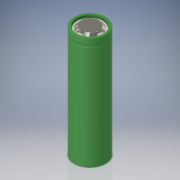
# Autodesk Inventor part: Battery18650
Saved by Autodesk Inventor 2017 (Build 210142000, 142)
## iProperties
Manager: Bradley
Company: Zetta & Zepto Technology
Created: 2016-08-15
Part Number: Battery18650
Material: Stainless Steel
Document SubType Name: Modeling
Designer: Bradley
Mass: 47 g
Surface Area: 43.2617 cm^2
Volume: 16.9329 cm^3
Density: 2.77566 g/cm^3
Appearance: Smooth - Dark Forest Green
Author: Bradley
Autodesk Inventor part; units mm, degrees
ref_plane "YZ Plane" through (0, 0, 0) normal (1, 0, 0) x (0, 1, 0)
ref_plane "XZ Plane" through (0, 0, 0) normal (0, 1, 0) x (-1, 0, 0)
ref_plane "XY Plane" through (0, 0, 0) normal (0, 0, 1) x (1, 0, 0)
sketch "Sketch1" plane through (0, 0, 0) normal (0, 0, 1) x (1, 0, 0)
  line L0 (0, 32.5) -> (0, -32.5)
  line L1 (9.15, -32.15) -> (9.15, 27.3)
  line L2 (9.15, 29.3) -> (9.15, 32)
  line L3 (8.85, 32.3) -> (7.95, 32.3)
  line L4 (7.65, 32) -> (7.65, 31.3)
  line L5 (7.35, 31) -> (6.65, 31)
  line L6 (6.65, 31) -> (5.2379, 32.4121)
  line L7 (5.0257, 32.5) -> (0, 32.5)
  arc A0 (8.85, -32.45) -> (9.15, -32.15) centre (8.85, -32.15) ccw
  arc A1 (9.15, 27.3) -> (9.0674, 27.5752) centre (8.65, 27.3) ccw
  arc A2 (9.0674, 29.0248) -> (9.15, 29.3) centre (8.65, 29.3) ccw
  arc A3 (9.15, 32) -> (8.85, 32.3) centre (8.85, 32) ccw
  arc A4 (5.2379, 32.4121) -> (5.0257, 32.5) centre (5.0257, 32.2) ccw
  arc A5 (7.95, 32.3) -> (7.65, 32) centre (7.95, 32) ccw
  arc A6 (7.35, 31) -> (7.65, 31.3) centre (7.35, 31.3) ccw
  arc A7 (9.0674, 29.0248) -> (9.0674, 27.5752) centre (10.1667, 28.3) ccw
  line L8 (8.85, -32.45) -> (8, -32.45)
  line L9 (0, -32.5) -> (8, -32.5)
  line L10 (8, -32.5) -> (8, -32.45)
  point P0 (0, 0)
  point P1 (9.15, 32.3)
  point P2 (7.65, 32.3)
  point P3 (7.65, 31)
  point P4 (0, 0)
  dimension "d0" = 65
  dimension "d1" = 18.3
  dimension "d2" = 0.2
  dimension "d3" = 1.5
  dimension "d4" = 1
  dimension "d5" = 135
  dimension "d6" = 1.3
  dimension "d9" = 0.3
  dimension "d19" = 0.3
  dimension "d20" = 0.5
  dimension "d21" = 4
  dimension "d22" = 2
  dimension "d23" = 0.05
  dimension "d24" = 16
  constraints: 22 end point, 16 point on circle, 14 tangent, 8 centre point, 7 point on line, 5 equal radius, 4 perpendicular, 2 horizontal, 1 coincident, 1 collinear, 1 midpoint, 1 vertical
  measures "d0" distance of L0.start L0.end
  measures "d1" diameter of L1 L0
  measures "d2" distance between parallel lines of L3 L7
  measures "d3" distance between parallel lines of L4 L2
  measures "d4" distance of point (7.65, 31) L5.end
  measures "d5" angle of L7 L6
  measures "d6" distance of point (7.65, 32.3) point (7.65, 31)
  measures "d9" radius of A0
  measures "d19" distance edge to line of A7 L2
  measures "d20" radius of A2
  measures "d21" distance from line of A7.centre L3
  measures "d22" distance of L1.end L2.start
  measures "d23" distance of L9.end L8.end
  measures "d24" diameter of L10 L0
revolve "Revolution1" add sketch "Sketch1" angle 360 about axis through (0, 32.5, 0) along (0, -1, 0)
sketch "Sketch2" plane through (0, 32.5, 0) normal (0, 1, 0) x (1, 0, 0)
  circle A0 centre (0, 0) radius 5.0257 projected
  circle A1 centre (0, 0) radius 7.35 projected
  circle A2 centre (0, 0) radius 7.65 projected
  circle A3 centre (0, 0) radius 7.65 projected
  circle A4 centre (0, 0) radius 7.65 projected
  circle A5 centre (0, 0) radius 7.65 projected
  line L0 (-2, -7.3839) -> (-2, -7.0257)
  line L1 (2, -7.0257) -> (2, -7.3839)
  arc A6 (2, -7.0257) -> (-2, -7.0257) centre (0, -7.0257) ccw
  circle A7 centre (0, 0) radius 7.35 projected
  arc A8 (-2, -7.0727) -> (2, -7.0727) centre (0, 0) ccw
  point P0 (0, 0)
  dimension "d11" = 4
  constraints: 8 point on circle, 4 end point, 3 tangent, 2 centre point, 2 point on line, 1 parallel, 1 vertical, 1 vertical alignment, 5 other
  measures "d11" distance between parallel lines of L0 L1
extrude "Extrusion2" cut sketch "Sketch2" against normal up to surface (1.5 mm away) contours A6 L1 A1 L0 picked at (0, -6.5546)
pattern_circular "Circular Pattern1" count 4 over 360 about axis through (0, -10, 0) along (0, 1, 0) of "Extrusion2"
body "Solid1"
